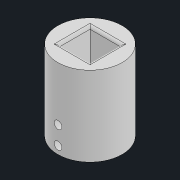
# Autodesk Inventor part: Motor-Driver Coupler
Saved by Autodesk Inventor 2022 (Build 260153000, 153)
## iProperties
Created: 2021-12-05
Part Number: Motor-Driver Coupler
Material: Generic
Document SubType Name: Modeling
Designer: alber
Density: 1 g/cm^3
Appearance: Default
Author: alber
Autodesk Inventor part; units mm, degrees
ref_plane "YZ Plane" through (0, 0, 0) normal (1, 0, 0) x (0, 1, 0)
ref_plane "XZ Plane" through (0, 0, 0) normal (0, 1, 0) x (-1, 0, 0)
ref_plane "XY Plane" through (0, 0, 0) normal (0, 0, 1) x (1, 0, 0)
ref_plane "Work Plane1" through (-82.8143, 19.6092, -42.8892) normal (0, 1, 0) x (0.9999998, 0, -0.0005571)
sketch "Sketch1" plane through (-82.8143, 19.6092, -42.8892) normal (0, 1, 0) x (0.9999998, 0, -0.0005571)
  arc A0 (1.5, -2) -> (-1.5, -2) centre (0, 0) ccw projected
  line L0 (-1.5, -2) -> (-1.1358, -2) projected
  line L1 (-1.1358, -2) -> (1.1358, -2) projected
  line L2 (1.1358, -2) -> (1.5, -2) projected
  line L3 (1.1358, -2.2) -> (-1.1358, -2.2)
  line L4 (-1.1358, -2.2) -> (-1.5652, -2.2)
  arc A1 (1.5652, -2.2) -> (-1.5652, -2.2) centre (0, 0) ccw
  line L5 (1.5652, -2.2) -> (1.1358, -2.2)
  circle A2 centre (0, 0) radius 12.5
  point P0 (82.7904, -42.9353)
  dimension "d0" = 0.2
  dimension "d1" = 25
  constraints: 6 end point, 2 centre point, 2 point on circle, 1 coincident, 3 other
  measures "d0" distance between parallel lines of L1 L3
  measures "d1" diameter of A2
extrude "Extrusion1" add sketch "Sketch1" against normal blind 13 contours A2
sketch "Sketch2" plane through (-81.2478, 6.6092, -40.69) normal (-0.0005571, 0, -0.9999998) x (-0.9999998, 0, 0.0005571)
  spline S0 degree 2 poles (3.0652, 12.8) (2.8756, 12.9138) (2.701, 13) knots 0 0 0 1 1 1 weights 1.078346 1.041437 1
  line L0 (3.0652, -2) -> (3.0652, 12.8)
  arc A0 (0.0652, -2) -> (3.0652, -2) centre (1.5652, 0.5981) ccw
  line L1 (0.0652, 12.8) -> (0.0652, -2)
  spline S1 degree 2 poles (0.4295, 13) (0.2549, 12.9138) (0.0652, 12.8) knots 0 0 0 1 1 1 weights 1 1.041437 1.078346
  line L2 (2.701, 13) -> (0.4295, 13)
  circle A1 centre (1.5652, 10) radius 1.5
  circle A2 centre (1.5652, 3) radius 1.5
  line L3 (-10.9348, 0) -> (14.0652, 0)
  point P0 (-81.2252, -6.6092)
  dimension "d4" = 3
  dimension "d5" = 3
  dimension "d6" = 3
  dimension "d7" = 3
  constraints: 2 centre point
  measures "d4" diameter of A1
  measures "d5" diameter of A2
  measures "d6" distance from line of L2 A1.centre
  measures "d7" distance from line of L3 A2.centre
extrude "Extrusion2" cut sketch "Sketch2" against normal blind 13 contours A1 | A2
sketch "Sketch3" plane through (-82.8143, 19.6092, -42.8892) normal (0, 1, 0) x (1, 0, 0)
  circle A0 centre (0, 0) radius 12.5 projected
  line L0 (1.5665, -2.1991) -> (-1.564, -2.2009) projected
  arc A1 (1.5665, -2.1991) -> (-1.564, -2.2009) centre (0, 0) ccw projected
  point P0 (82.8143, -42.8892)
extrude "Extrusion3" add sketch "Sketch3" along normal blind 3 contours A0 | L0 A1
move faces "Move1" translate (0, 15, 0) faces at (-80.4474, 22.6092, -41.4544)
sketch "Sketch5" plane through (-82.8143, 37.6092, -42.8892) normal (0, 1, 0) x (1, 0, 0)
  line L0 (6, 6) -> (-6, 6)
  line L1 (-6, 6) -> (-6, -6)
  line L2 (-6, -6) -> (6, -6)
  line L3 (6, -6) -> (6, 6)
  line L4 (6, 6) -> (-6, -6) construction
  line L5 (-6, 6) -> (6, -6) construction
  point P0 (82.8143, -42.8892)
  point P1 (0, 0)
  dimension "d18" = 12
  dimension "d19" = 12
  constraints: 12 end point, 2 midpoint, 2 parallel, 1 horizontal, 1 perpendicular
  measures "d18" distance of L2.end L1.end
  measures "d19" distance of L1.end L0.end
extrude "Extrusion5" cut sketch "Sketch5" against normal blind 20
fillet "Fillet2" radius 1 4 edges at (-82.8143, 37.6092, -36.8892) (-76.8143, 37.6092, -42.8892) (-82.8143, 37.6092, -48.8892) (-88.8143, 37.6092, -42.8892)
sketch "Sketch6" plane through (-82.8143, 17.6092, -42.8892) normal (0, 1, 0) x (1, 0, 0)
  line L0 (-1.1168, -2.2006) -> (-1.1147, -6) projected
  line L1 (-1.564, -2.2009) -> (-1.1168, -2.2006) projected
  arc A0 (1.5665, -2.1991) -> (-1.564, -2.2009) centre (0, 0) ccw projected
  line L2 (1.1193, -2.1994) -> (1.5665, -2.1991) projected
  line L3 (1.1214, -6) -> (1.1193, -2.1994) projected
  line L4 (6, -6) -> (1.1214, -6) projected
  line L5 (6, 6) -> (6, -6) projected
  line L6 (-6, 6) -> (6, 6) projected
  line L7 (-6, -6) -> (-6, 6) projected
  line L8 (-1.1147, -6) -> (-6, -6) projected
  line L9 (6, -6) -> (-6, -6) projected
equation "\"d7\" = d6"
body "Solid1"
